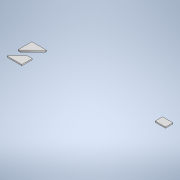
# Autodesk Inventor part: BungaSign-Bigger-Seams
Saved by Autodesk Inventor 2022 (Build 260153000, 153)
## iProperties
Created: 2022-08-11
Part Number: BungaSign-Bigger-Seams
Material: Generic
Document SubType Name: Modeling
Designer: incep
Density: 1 g/cm^3
Appearance: Default
Author: incep
Autodesk Inventor part; units mm, degrees
ref_plane "YZ Plane" through (0, 0, 0) normal (1, 0, 0) x (0, 1, 0)
ref_plane "XZ Plane" through (0, 0, 0) normal (0, 1, 0) x (-1, 0, 0)
ref_plane "XY Plane" through (0, 0, 0) normal (0, 0, 1) x (1, 0, 0)
sketch "Sketch1" plane through (0, 0, 0) normal (0, 1, 0) x (-1, 0, 0)
  line L0 (254, -152.4) -> (-254, -152.4) construction
  line L1 (-254, -152.4) -> (-254, 152.4) construction
  line L2 (-254, 152.4) -> (254, 152.4) construction
  line L3 (254, 152.4) -> (254, -152.4) construction
  line L4 (250, -150) -> (-250, -150) construction
  line L5 (-250, -150) -> (-250, 150) construction
  line L6 (-250, 150) -> (250, 150) construction
  line L7 (250, 150) -> (250, -150) construction
  line L8 (35, -51) -> (-35, -51) construction
  line L9 (-35, -51) -> (-35, 51) construction
  line L10 (-35, 51) -> (35, 51) construction
  line L11 (35, 51) -> (35, -51) construction
  line L12 (-52, -51) -> (-122, -51) construction
  line L13 (-52, 51) -> (-52, -51) construction
  line L14 (-122, 51) -> (-52, 51) construction
  line L15 (-122, -51) -> (-122, 51) construction
  line L16 (-139, -51) -> (-209, -51) construction
  line L17 (-139, 51) -> (-139, -51) construction
  line L18 (-209, 51) -> (-139, 51) construction
  line L19 (-209, -51) -> (-209, 51) construction
  line L20 (122, -51) -> (52, -51) construction
  line L21 (122, 51) -> (122, -51) construction
  line L22 (52, 51) -> (122, 51) construction
  line L23 (52, -51) -> (52, 51) construction
  line L24 (35, -51) -> (-35, -51) construction
  line L25 (35, 51) -> (35, -51) construction
  line L26 (-35, 51) -> (35, 51) construction
  line L27 (-35, -51) -> (-35, 51) construction
  line L28 (-52, -51) -> (-122, -51) construction
  line L29 (-52, 51) -> (-52, -51) construction
  line L30 (-122, 51) -> (-52, 51) construction
  line L31 (-122, -51) -> (-122, 51) construction
  line L32 (209, -51) -> (139, -51) construction
  line L33 (209, 51) -> (209, -51) construction
  line L34 (139, 51) -> (209, 51) construction
  line L35 (139, -51) -> (139, 51) construction
  line L36 (122, -51) -> (52, -51) construction
  line L37 (122, 51) -> (122, -51) construction
  line L38 (52, 51) -> (122, 51) construction
  line L39 (52, -51) -> (52, 51) construction
  line L40 (35, -51) -> (-35, -51) construction
  line L41 (35, 51) -> (35, -51) construction
  line L42 (-35, 51) -> (35, 51) construction
  line L43 (-35, -51) -> (-35, 51) construction
  line L44 (35, 51) -> (35, -51)
  line L45 (35, -51) -> (-7, -51)
  line L46 (-7, -51) -> (-7, 17)
  line L47 (-7, 17) -> (-21, 31)
  line L48 (-21, 31) -> (-21, -51)
  line L49 (-21, -51) -> (-35, -51)
  line L50 (-35, -51) -> (-35, 51)
  line L51 (-35, 51) -> (7, 51)
  line L52 (7, 51) -> (7, -22)
  line L53 (7, -22) -> (21, -36)
  line L54 (21, -36) -> (21, 51)
  line L55 (21, 51) -> (35, 51)
  line L56 (0, -51) -> (0, 51) construction
  line L57 (-122, -51) -> (-52, -51)
  line L58 (-52, -51) -> (-52, 51)
  line L59 (-52, 51) -> (-122, 51)
  line L60 (-122, 51) -> (-122, -21)
  line L61 (-122, -21) -> (-96, -21)
  line L62 (-96, -21) -> (-96, -6)
  line L63 (-96, -6) -> (-107, -6)
  line L64 (-107, -6) -> (-107, 31)
  line L65 (-107, 31) -> (-67, 31)
  line L66 (-67, 31) -> (-67, -36)
  line L67 (-67, -36) -> (-122, -36)
  line L68 (-122, -36) -> (-122, -51)
  line L69 (-139, 51) -> (-160, 51)
  line L70 (-160, 51) -> (-160, -2)
  line L71 (-160, -2) -> (-188, -2)
  line L72 (-188, -2) -> (-188, 51)
  line L73 (-188, 51) -> (-209, 51)
  line L74 (-209, 51) -> (-209, -51)
  line L75 (-209, -51) -> (-139, -51)
  line L76 (-139, -51) -> (-139, 51)
  line L77 (-160, -37) -> (-160, -17)
  line L78 (-160, -17) -> (-188, -17)
  line L79 (-188, -17) -> (-188, -37)
  line L80 (-188, -37) -> (-160, -37)
  line L81 (122, -51) -> (105, -51)
  line L82 (105, -51) -> (105, 31)
  line L83 (105, 31) -> (69, 31)
  line L84 (69, 31) -> (69, -51)
  line L85 (69, -51) -> (52, -51)
  line L86 (52, -51) -> (52, 51)
  line L87 (52, 51) -> (122, 51)
  line L88 (122, 51) -> (122, -51)
  line L89 (209, -51) -> (209, 51)
  line L90 (209, 51) -> (139, 51)
  line L91 (139, -51) -> (209, -51)
  line L92 (194, -36) -> (194, 1.1241)
  line L93 (194, -17.438) -> (166.3593, -17.438) construction
  line L94 (149.2402, 0) -> (139, 0) construction
  line L95 (194, 1.1241) -> (188.5027, 1.1241)
  line L96 (188.5027, 1.1241) -> (154, -33.3786)
  line L97 (188.5027, 1.1241) -> (237.2968, 1.1241) construction
  line L98 (154, -33.3786) -> (154, -36)
  line L99 (154, -36) -> (194, -36)
  line L100 (149.2402, 0) -> (139, 0)
  line L101 (169, 2.9543) -> (154, 2.9543)
  line L102 (154, 2.9543) -> (154, 31)
  line L103 (154, 31) -> (194, 31)
  line L104 (194, 31) -> (194, 27.9543)
  line L105 (194, 27.9543) -> (169, 2.9543)
  line L106 (194, 27.9543) -> (222.5108, 27.9543) construction
  line L107 (232, -74) -> (-232, -74) construction
  line L108 (-232, -74) -> (-232, 74)
  line L109 (-232, 74) -> (232, 74)
  line L110 (232, 74) -> (232, -74)
  line L111 (139, -51) -> (139, -27.0457)
  line L112 (139, -27.0457) -> (154, -12.0457)
  line L113 (139, -27.0457) -> (160.2132, -27.0457) construction
  line L114 (154, -12.0457) -> (139, -12.0457)
  line L115 (139, 51) -> (139, -12.0457)
  line L116 (154, -12.0457) -> (169, 2.9543) construction
  circle A0 centre (0, -56) radius 1.85
  circle A1 centre (107, -56) radius 1.85
  circle A2 centre (-107, -56) radius 1.85
  circle A3 centre (107, 56) radius 1.85
  circle A4 centre (-107, 56) radius 1.85
  circle A5 centre (0, 56) radius 1.85
  circle A6 centre (214, -56) radius 1.85
  circle A7 centre (214, 56) radius 1.85
  circle A8 centre (-214, 56) radius 1.85
  circle A9 centre (-214, -56) radius 1.85
  line L117 (232, -74) -> (222.1, -74)
  line L118 (222.1, -74) -> (222.1, -71.05)
  line L119 (222.1, -71.05) -> (212.2, -71.05)
  line L120 (212.2, -71.05) -> (212.2, -74)
  point P0 (0, 0)
  point P1 (254, 0)
  point P2 (0, -152.4)
  point P3 (0, -150)
  point P4 (-250, 0)
  point P5 (-40, 0)
  point P6 (0, -80)
  point P7 (0, -51)
  point P8 (-35, 0)
  point P9 (-87, -51)
  point P10 (-87, 0)
  point P11 (-122, 0)
  point P12 (-174, -51)
  point P13 (-174, 0)
  point P14 (-209, 0)
  point P15 (87, -51)
  point P16 (87, 0)
  point P17 (52, 0)
  point P18 (0, -51)
  point P19 (0, 0)
  point P20 (-35, 0)
  point P21 (-87, -51)
  point P22 (-87, 0)
  point P23 (-122, 0)
  point P24 (174, -51)
  point P25 (174, 0)
  point P26 (139, 0)
  point P27 (87, -51)
  point P28 (87, 0)
  point P29 (52, 0)
  point P30 (0, 0)
  point P31 (-35, 0)
  point P32 (149.2402, 0)
  point P33 (128.5, -20.7402)
  point P34 (-232, 0)
  point P35 (0, 0)
  point P36 (0, -74)
  point P37 (192.2235, 31)
  dimension "d0" = 508
  dimension "d1" = 304.8
  dimension "d2" = 500
  dimension "d3" = 300
  dimension "d6" = 70
  dimension "d7" = 102
  dimension "d10" = 87
  dimension "d13" = 87
  dimension "d16" = 135
  dimension "d17" = 135
  dimension "d18" = 14
  dimension "d19" = 14
  dimension "d20" = 15
  dimension "d21" = 20
  dimension "d22" = 15
  dimension "d23" = 15
  dimension "d24" = 20
  dimension "d25" = 15
  dimension "d26" = 15
  dimension "d27" = 11
  dimension "d28" = 15
  dimension "d29" = 21
  dimension "d30" = 21
  dimension "d31" = 14
  dimension "d32" = 20
  dimension "d33" = 15
  dimension "d34" = 17
  dimension "d35" = 20
  dimension "d36" = 17
  dimension "d43" = 0
  dimension "d45" = 15
  dimension "d47" = 135
  dimension "d49" = 15
  dimension "d51" = 135
  dimension "d56" = 20
  dimension "d57" = 45
  dimension "d58" = 15
  dimension "d59" = 15
  dimension "d62" = 45
  dimension "d63" = 464
  dimension "d64" = 15
  dimension "d67" = 148
  dimension "d68" = 418
  dimension "d69" = 102
  dimension "d70" = 14
  dimension "d71" = 3.7
  dimension "d72" = 5
  dimension "d73" = 5
  dimension "d74" = 107
  dimension "d75" = 107
  dimension "d76" = 107
  dimension "d77" = 107
  dimension "d78" = 9.9
  dimension "d79" = 2.95
  dimension "d80" = 9.9
  constraints: 242 end point, 33 perpendicular, 20 point on line, 18 collinear, 15 horizontal alignment, 13 horizontal, 12 midpoint, 11 vertical alignment, 10 centre point, 10 parallel, 9 equal radius, 6 vertical, 2 equal length, 1 coincident, 92 other
  measures "d0" distance of L0.start L0.end
  measures "d1" distance of L2.end L0.start
  measures "d2" distance of L4.start L4.end
  measures "d3" distance of L6.end L4.start
  measures "d6" distance of L8.start L8.end
  measures "d7" distance of L10.end L8.start
  measures "d10" distance of point (0, -51) point (-87, -51)
  measures "d13" distance of point (0, -51) point (87, -51)
  measures "d16" angle of L47 L46
  measures "d17" angle of L53 L52
  measures "d18" distance between parallel lines of L54 L11
  measures "d19" distance between parallel lines of L46 L52
  measures "d20" vertical distance of point (0, -51) L53.end
  measures "d21" distance from line of L10 L47.end
  measures "d22" distance of L67.end L28.end
  measures "d23" distance between parallel lines of L66 L29
  measures "d24" distance between parallel lines of L14 L65
  measures "d25" distance of L61.end L62.end
  measures "d26" distance between parallel lines of L67 L61
  measures "d27" distance of L62.end L63.end
  measures "d28" distance between parallel lines of L15 L64
  measures "d29" distance of L17.start L69.end
  measures "d30" distance of L72.end L18.start
  measures "d31" distance between parallel lines of L16 L80
  measures "d32" distance of L78.end L79.end
  measures "d33" distance between parallel lines of L71 L78
  measures "d34" distance between parallel lines of L82 L21
  measures "d35" distance between parallel lines of L22 L83
  measures "d36" distance between parallel lines of L23 L84
  measures "d43" distance of point (149.24, 0) L100.start
  measures "d45" distance between parallel lines of L33 L92
  measures "d47" angle of L96 L97
  measures "d49" distance between parallel lines of L91 L99
  measures "d51" angle of L105 L106
  measures "d56" distance between parallel lines of L34 L103
  measures "d57" angle of L113 L112
  measures "d58" distance between parallel lines of L114 L101
  measures "d59" distance between parallel lines of L35 L98
  measures "d62" angle of L116 L101
  measures "d63" distance of L107.start L107.end
  measures "d64" distance of L112.end L114.end
  measures "d67" distance of L109.end L107.start
  measures "d68" distance between parallel lines of L19 L33
  measures "d69" distance of L32.start L33.start
  measures "d70" distance between parallel lines of L9 L48
  measures "d71" diameter of A0
  measures "d72" distance from line of A0.centre L8
  measures "d73" distance from line of L10 A5.centre
  measures "d74" distance of A0.centre A1.centre
  measures "d75" distance of A2.centre A0.centre
  measures "d76" distance of A6.centre A1.centre
  measures "d77" distance of A9.centre A2.centre
  measures "d78" distance of L107.start L117.end
  measures "d79" distance of L117.end L118.end
  measures "d80" distance of L118.end L119.end
extrude "Extrusion2" add sketch "Sketch1" along normal blind 3 contours L80 L79 L78 L77 | L99 L98 L96 L95 L92 | L101 L102 L103 L104 L105
equation "\"kerf\" = 0.1"
equation "\"thickness\" = 3"
body "Solid2"
